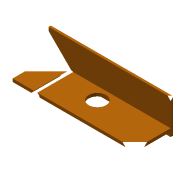
# Autodesk Inventor part: P_hips02_001
Saved by Autodesk Inventor 2016 (Build 200138000, 138)
## iProperties
Created: 2016-02-25
Part Number: P_hips02_001
Material: PC/ABS Plastic
Document SubType Name: Modeling
Designer: Mateusz
Density: 0.357273 g/cm^3
Appearance: Orange
Author: Mateusz
Autodesk Inventor part; units mm, degrees
ref_plane "YZ Plane" through (0, 0, 0) normal (1, 0, 0) x (0, 1, 0)
ref_plane "XY Plane" through (0, 0, 0) normal (0, 0, 1) x (1, 0, 0)
derived "skeleton.ipt"
sketch "Sketch1" plane through (0, 0, 0) normal (0, 0, 1) x (1, 0, 0)
  line L0 (0, -37.5) -> (150, -37.5)
  line L1 (150, -37.5) -> (150, 37.5)
  line L2 (150, 37.5) -> (0, 37.5)
  line L3 (0, 37.5) -> (0, -37.5)
  line L4 (0, -56) -> (0, 56) projected
  line L5 (-32, 0) -> (192, 0) projected
  point P0 (0, 0)
  dimension "d1" = 150
  dimension "d2" = 75
  constraints: 8 end point, 2 parallel, 1 collinear, 1 horizontal, 1 perpendicular, 1 other
  measures "d1" distance between parallel lines of L3 L1
  measures "d2" distance between parallel lines of L0 L2
extrude "Extrusion1" add sketch "Sketch1" along normal blind 3
ref_plane "Work Plane1" through (0, 1, 0) normal (0, 1, 0) x (-1, 0, 0)
sketch "Sketch3" plane through (0, 1, 0) normal (0, 1, 0) x (-1, 0, 0)
  line L0 (0, -10) -> (0, 60) projected
  line L1 (32, 0) -> (-192, 0) projected
  line L2 (0, 0) -> (-150, 0)
  line L3 (-150, 0) -> (-150, 50)
  line L4 (-150, 50) -> (0, 50)
  line L5 (0, 50) -> (0, 0)
  dimension "d10" = 150
  dimension "d11" = 50
  constraints: 8 end point, 2 parallel, 1 horizontal, 1 perpendicular
  measures "d10" distance between parallel lines of L3 L5
  measures "d11" distance between parallel lines of L4 L1
extrude "Extrusion3" add sketch "Sketch3" along normal blind 4
sketch "Sketch4" plane through (0, -37.5, 0) normal (0, -1, 0) x (1, 0, 0)
  line L0 (0, 60) -> (0, -10) projected
  line L1 (-31.6851, 0) -> (190.1108, 0) projected
  line L2 (88.4257, 19) -> (158.4257, 19)
  point P0 (0, 0)
  point P1 (90, 19)
  dimension "d14" = 90
  constraints: 2 end point, 1 horizontal, 1 point on line, 2 other
  measures "d14" distance from line of point (90, 19) L0
hole "Hole1" at (90, -37.5, 19) direction (0, 1, 0) diameter 23 end through all
sketch "Sketch5" plane through (0, 0, 0) normal (0, 0, 1) x (1, 0, 0)
  line L0 (-6, 0) -> (36, 0) projected
  line L1 (0, -21) -> (0, 21) projected
  point P0 (0, 0)
  point P1 (30, 0)
  dimension "d22" = 30
  constraints: 1 point on line
  measures "d22" distance from line of L1 point (30, 0)
hole "Hole2" at (30, 0, 0) direction (0, 0, 1) diameter 11 end through all
sketch "Sketch6" plane through (0, 0, 0) normal (0, 0, 1) x (1, 0, 0)
  line L0 (-32, 0) -> (192, 0) projected
  line L1 (0, 9.2) -> (0, -48.2) projected
  line L2 (150, -37.5) -> (0, -37.5)
  line L3 (0, -37.5) -> (0, 1)
  line L4 (0, 1) -> (150, 1)
  line L5 (150, 1) -> (150, -37.5)
  point P0 (0, 0)
  dimension "d31" = 37.5
  dimension "d32" = 0
  dimension "d33" = 150
  dimension "d37" = 1
  constraints: 8 end point, 2 parallel, 1 horizontal, 1 perpendicular
  measures "d31" distance between parallel lines of L0 L2
  measures "d32" distance between parallel lines of L1 L3
  measures "d33" distance between parallel lines of L1 L5
  measures "d37" distance between parallel lines of L4 L0
extrude "Extrusion4" cut sketch "Sketch6" along normal blind 3
sketch "Sketch8" plane through (0, 0, 0) normal (0, 0, 1) x (1, 0, 0)
  line L0 (0, 48) -> (0, -8) projected
  line L1 (-32, 0) -> (192, 0) projected
  line L2 (150, 37.5) -> (0, 37.5) projected
  line L3 (0, 37.5) -> (0, 5) projected
  line L4 (50, 0) -> (50, 37.5)
  point P0 (0, 0)
  dimension "d38" = 50
  constraints: 2 end point, 2 point on line, 1 vertical
  measures "d38" distance between parallel lines of L0 L4
extrude "Extrusion5" cut sketch "Sketch8" along normal through all
sketch "Sketch9" plane through (0, 5, 0) normal (0, 1, 0) x (1, 0, 0)
  arc A0 (58.5256, -31.9896) -> (60.4744, -31.9896) centre (59.5, -32.5) ccw projected
  arc A1 (66.5256, -31.9896) -> (68.4744, -31.9896) centre (67.5, -32.5) ccw projected
  circle A2 centre (75.5, -32.5) radius 1.1 projected
  arc A3 (82.5256, -31.9896) -> (84.4744, -31.9896) centre (83.5, -32.5) ccw projected
  arc A4 (54.5104, -26.0256) -> (54.5104, -27.9744) centre (54, -27) ccw projected
  circle A5 centre (54, -11) radius 1.1 projected
  circle A6 centre (59.5, -5.5) radius 1.1 projected
  circle A7 centre (67.5, -5.5) radius 1.1 projected
  circle A8 centre (75.5, -5.5) radius 1.1 projected
  circle A9 centre (83.5, -5.5) radius 1.1 projected
  point P0 (0, 0)
hole "Hole3" at (83.5, 5, 32.5) at (75.5, 5, 32.5) at (67.5, 5, 32.5) at (59.5, 5, 32.5) at (54, 5, 27) at (54, 5, 11) at (59.5, 5, 5.5) at (67.5, 5, 5.5) at (75.5, 5, 5.5) at (83.5, 5, 5.5) direction (0, -1, 0) diameter 2.6 end through all
chamfer "Chamfer1" distance 1 angle 45 10 edges at (83.5, 1, 31.2) (75.5, 1, 31.2) (67.5, 1, 31.2) (59.5, 1, 31.2) (54, 1, 25.7) (54, 1, 9.7) (59.5, 1, 4.2) (67.5, 1, 4.2) (75.5, 1, 4.2) (83.5, 1, 4.2)
equation "\"d1\" = 0.5 * hips_width"
equation "\"d2\" = hips_length"
equation "\"d10\" = 0.5 * hips_width"
equation "\"d14\" = 0.5 * arm_spc"
equation "\"d22\" = 0.5 * leg_spc"
equation "\"d31\" = 0.5 * hips_length"
equation "\"d33\" = 0.5 * hips_width"
equation "\"wall\" = 3"
equation "\"hips_width\" = 300"
equation "\"hips_length\" = 75"
equation "\"arm_spc\" = 180"
equation "\"leg_spc\" = 60"
body "Solid1"
